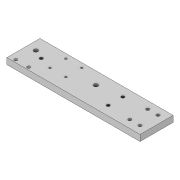
# Autodesk Inventor part: Columna Derecha
Saved by Autodesk Inventor 2020 (Build 240168000, 168)
## iProperties
Created: 2020-05-17
Part Number: Columna Derecha
Material: Aluminio 6061
Document SubType Name: Modeling
Designer: Pipi
Density: 2.7 g/cm^3
Appearance: Aluminum - Dark
Mass: 192.235 g
Surface Area: 470.037 cm^2
Volume: 192.235 cm^3
Author: Pipi
Autodesk Inventor part; units mm, degrees
ref_plane "YZ Plane" through (0, 0, 0) normal (1, 0, 0) x (0, 1, 0)
ref_plane "XZ Plane" through (0, 0, 0) normal (0, 1, 0) x (-1, 0, 0)
ref_plane "XY Plane" through (0, 0, 0) normal (0, 0, 1) x (1, 0, 0)
sketch "Boceto1" plane through (0, 0, 0) normal (0, 1, 0) x (-1, 0, 0)
  line L0 (6.1283, -21.2541) -> (6.1283, -85.7541)
  line L1 (6.1283, -85.7541) -> (-253.3717, -85.7541)
  line L2 (6.1283, -21.2541) -> (-253.3717, -21.2541)
  line L3 (-253.3717, -21.2541) -> (-253.3717, -85.7541)
  circle A0 centre (-127.3717, -61.2541) radius 4
  circle A1 centre (-10.3717, -61.2541) radius 4
  circle A2 centre (-84.3717, -76.7541) radius 2
  circle A3 centre (-84.3717, -45.7541) radius 2
  circle A4 centre (-53.3717, -76.7541) radius 2
  circle A5 centre (-53.3717, -45.7541) radius 2
  circle A6 centre (-28.8717, -53.2541) radius 3
  circle A7 centre (-173.3717, -67.7541) radius 3
  circle A8 centre (-173.3717, -39.2541) radius 3
  dimension "d0" = 64.5
  dimension "d22" = 8
  dimension "d23" = 8
  dimension "d65" = 4
  dimension "d66" = 4
  dimension "d67" = 4
  dimension "d68" = 4
  dimension "d69" = 31
  dimension "d70" = 31
  dimension "d71" = 31
  dimension "d72" = 31
  dimension "d109" = 117
  dimension "d110" = 259.5
  dimension "d111" = 126
  dimension "d112" = 6
  dimension "d113" = 32
  dimension "d114" = 35
  dimension "d115" = 6
  dimension "d116" = 6
  dimension "d117" = 18
  dimension "d118" = 18
  dimension "d119" = 80
  dimension "d120" = 80
  dimension "d127" = 40
  dimension "d128" = 40
  constraints: 9 centre point, 8 end point, 2 perpendicular, 1 horizontal, 1 vertical
  measures "d0" distance of L0.start L0.end
  measures "d22" diameter of A0
  measures "d23" diameter of A1
  measures "d65" diameter of A2
  measures "d66" diameter of A3
  measures "d67" diameter of A4
  measures "d68" diameter of A5
  measures "d69" distance of A4.centre A5.centre
  measures "d70" distance of A2.centre A3.centre
  measures "d71" distance of A2.centre A4.centre
  measures "d72" distance of A3.centre A5.centre
  measures "d109" distance of A1.centre A0.centre
  measures "d110" distance of L0.end L1.end
  measures "d111" distance from line of A0.centre L3
  measures "d112" diameter of A6
  measures "d113" distance from line of L2 A6.centre
  measures "d114" distance from line of L0 A6.centre
  measures "d115" diameter of A7
  measures "d116" diameter of A8
  measures "d117" distance from line of L1 A7.centre
  measures "d118" distance from line of L2 A8.centre
  measures "d119" distance from line of L3 A7.centre
  measures "d120" distance from line of L3 A8.centre
  measures "d127" distance from line of L2 A1.centre
  measures "d128" distance from line of L2 A0.centre
extrude "Extrusion3" add sketch "Boceto1" along normal blind 12
sketch "Sketch2" plane through (0, 0, 0) normal (0, -1, 0) x (1, 0, 0)
  circle A0 centre (6.3717, -26.2541) radius 3
  circle A1 centre (31.3717, -26.2541) radius 3
  line L0 (-6.1283, -21.2541) -> (253.3717, -21.2541) projected
  line L1 (-6.1283, -85.7541) -> (-6.1283, -21.2541) projected
  point P0 (0, 0)
  point P1 (-7.1283, -20.7541)
  point P2 (261.8717, -20.7541)
  point P3 (-7.1283, -85.7541)
  dimension "d84" = 6
  dimension "d85" = 6
  dimension "d86" = 5
  dimension "d87" = 12.5
  dimension "d88" = 25
  dimension "d89" = 5
  constraints: 2 centre point, 2 other
  measures "d84" diameter of A0
  measures "d85" diameter of A1
  measures "d88" distance of A1.centre A0.centre
extrude "Extrusion4" cut sketch "Sketch2" against normal blind 19
sketch "Sketch3" plane through (0, 12, 0) normal (0, 1, 0) x (1, 0, 0)
  circle A0 centre (218.3717, 71.2541) radius 3
  circle A1 centre (238.3717, 71.2541) radius 3
  circle A2 centre (218.3717, 36.2541) radius 3
  circle A3 centre (238.3717, 36.2541) radius 3
  line L0 (253.3717, 85.7541) -> (-6.1283, 85.7541) projected
  line L1 (-6.1283, 21.2541) -> (253.3717, 21.2541) projected
  line L2 (253.3717, 21.2541) -> (253.3717, 85.7541) projected
  point P0 (-7.1283, 85.7541)
  point P1 (-7.1283, 20.7541)
  dimension "d92" = 6
  dimension "d93" = 6
  dimension "d94" = 6
  dimension "d95" = 6
  dimension "d97" = 15
  dimension "d98" = 15
  dimension "d99" = 15
  dimension "d100" = 20
  dimension "d101" = 20
  dimension "d103" = 15
  dimension "d130" = 35
  dimension "d131" = 35
  constraints: 4 centre point, 1 other
  measures "d92" diameter of A0
  measures "d93" diameter of A1
  measures "d94" diameter of A2
  measures "d95" diameter of A3
  measures "d98" distance from line of A1.centre L2
  measures "d99" distance from line of A3.centre L2
  measures "d100" distance of A0.centre A1.centre
  measures "d101" distance of A2.centre A3.centre
  measures "d130" distance of A2.centre A0.centre
  measures "d131" distance of A3.centre A1.centre
extrude "Extrusion5" cut sketch "Sketch3" against normal blind 20
thread "Rosca1" size "M6x1" class "6H" standard "ISO Metric profile" length 922
thread "Rosca2" size "M6x1" class "6H" standard "ISO Metric profile" length 922
thread "Rosca3" size "M6x1" class "6H" standard "ISO Metric profile" length 922
equation "\"d22\" = d23"
equation "\"d118\" = d117"
equation "\"d120\" = d119"
equation "\"d131\" = d130"
equation "\"d104\" = d100"
body "Solid3"
